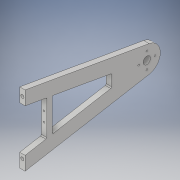
# Autodesk Inventor part: halter_seite
Saved by Autodesk Inventor 2017 (Build 210142000, 142)
## iProperties
Part Number: halter_seite
Material: Generisch
Document SubType Name: Modeling
Designer: Fabio
Density: 1 g/cm^3
Appearance: Vorgabe
Author: Fabio
Autodesk Inventor part; units mm, degrees
ref_plane "YZ Plane" through (0, 0, 0) normal (1, 0, 0) x (0, 1, 0)
ref_plane "XZ Plane" through (0, 0, 0) normal (0, 1, 0) x (-1, 0, 0)
ref_plane "XY Plane" through (0, 0, 0) normal (0, 0, 1) x (1, 0, 0)
sketch "Skizze1" plane through (0, 0, 0) normal (1, 0, 0) x (0, 1, 0)
  arc A0 (250, 65.0592) -> (229.3412, 89.6794) centre (225, 65.0592) ccw
  line L0 (225, 65.0592) -> (229.3412, 89.6794) construction
  line L1 (225, 65.0592) -> (250, 65.0592) construction
  line L2 (229.3412, 89.6794) -> (0, 130.1185)
  line L3 (0, 130.1185) -> (0, 104.7328)
  arc A1 (229.3412, 40.439) -> (250, 65.0592) centre (225, 65.0592) ccw
  line L4 (229.3412, 40.439) -> (0, 0)
  line L5 (0, 0) -> (92.864, 0) construction
  line L6 (0, 0) -> (0, 25.3857)
  line L7 (160, 76.5205) -> (160, 53.598)
  line L8 (40, 97.6797) -> (40, 32.4387)
  line L9 (50, 34.202) -> (50, 95.9165)
  line L10 (0, 104.7328) -> (40, 97.6797)
  line L11 (50, 95.9165) -> (160, 76.5205)
  line L12 (0, 25.3857) -> (40, 32.4387)
  line L13 (50, 34.202) -> (160, 53.598)
  dimension "d21" = 80
  dimension "d24" = 25
  dimension "d68" = 250
  dimension "d73" = 80
  dimension "d88" = 130.1185
  dimension "d89" = 79.3471
  dimension "d91" = 10
  dimension "d92" = 25
  dimension "d93" = 25
  dimension "d94" = 40
  dimension "d96" = 25
  dimension "d97" = 25
  dimension "d127" = 110
  constraints: 28 end point, 4 point on circle, 4 vertical, 2 centre point, 2 parallel, 2 symmetric about line, 1 coincident, 1 horizontal, 1 other
  measures "d21" angle of L1 L0
  measures "d24" radius of A0
  measures "d68" distance from line of L1.end L3
  measures "d73" angle of L3 L2
  measures "d88" distance of point (0, 0) L2.end
  measures "d89" distance of L6.end L3.end
  measures "d91" distance between parallel lines of L8 L9
  measures "d92" distance between parallel lines of L2 L11
  measures "d93" distance between parallel lines of L4 L13
  measures "d94" distance from line of L8 L3.end
  measures "d96" distance between parallel lines of L2 L10
  measures "d97" distance between parallel lines of L4 L12
  measures "d127" distance between parallel lines of L9 L7
extrude "Extrusion2" add sketch "Skizze1" along normal blind 10
sketch "Skizze7" plane through (10, 0, 0) normal (1, 0, 0) x (0, 0, -1)
  arc A0 (-40.439, 229.3412) -> (-89.6794, 229.3412) centre (-65.0592, 225) ccw projected
  point P0 (0, 0)
  constraints: 1 coincident
hole "Bohrung6" at (10, 225, 65.0592) direction (-1, 0, 0) diameter 13.6 end through all
sketch "Skizze8" plane through (10, 0, 0) normal (1, 0, 0) x (0, 0, -1)
  circle A0 centre (-65.0592, 225) radius 6.8 projected
  line L0 (-65.0592, 225) -> (-65.0592, 240) construction
  point P0 (0, 0)
  point P1 (-80.0592, 225)
  point P2 (-65.0592, 210)
  point P3 (-50.0592, 225)
  dimension "d107" = 15
  dimension "d110" = 360
  constraints: 2 end point, 1 coincident, 1 vertical, 5 other
  measures "d107" distance of L0.start L0.end
hole "Bohrung7" at (10, 240, 65.0592) at (10, 225, 80.0592) at (10, 210, 65.0592) at (10, 225, 50.0592) direction (-1, 0, 0) diameter 3 end through all
sketch "Skizze9" plane through (0, 0, 104.7328) normal (0, -1, 0) x (1, 0, 0)
  line L0 (0, 25.3857) -> (10, 25.3857) construction
  line L1 (5, 25.3857) -> (5, -104.7328) construction
  line L2 (0, -104.7328) -> (10, -104.7328) construction
  line L3 (0, 25.3857) -> (0, 0) construction
  line L4 (10, 25.3857) -> (10, 0) construction
  line L5 (0, 25.3857) -> (0, 0) construction
  line L6 (0, 0) -> (10, 0) construction
  line L7 (10, 25.3857) -> (10, 0) construction
  line L8 (0, 25.3857) -> (10, 25.3857) construction
  line L9 (0, 12.6928) -> (10, 12.6928) construction
  point P0 (5, 12.6928)
  point P1 (5, -87.3072)
  dimension "d119" = 100
  constraints: 5 midpoint, 4 end point, 1 point on line
  measures "d119" distance of point (5, 12.693) point (5, -87.307)
hole "Bohrung8" at (5, 0, 117.4256) at (5, 0, 17.4256) direction (0, 1, 0) diameter 6 depth 20 tip angle 118
sketch "Skizze10" plane through (0, 50, 95.9165) normal (0, 1, 0) x (1, 0, 0)
  line L0 (10, 61.7144) -> (10, 0) construction
  line L1 (10, 30.8572) -> (0, 30.8572) construction
  point P0 (0, 95.9165)
  point P1 (5, 21.8572)
  point P2 (5, 39.8572)
  dimension "d128" = 5
  dimension "d130" = 9
  dimension "d132" = 5
  dimension "d133" = 18
  constraints: 2 end point, 1 horizontal, 1 midpoint
  measures "d128" distance from line of point (5, 21.857) L0
  measures "d130" distance from line of L1 point (5, 21.857)
  measures "d132" distance from line of L0 point (5, 39.857)
  measures "d133" distance of point (5, 39.857) point (5, 21.857)
hole "Bohrung9" at (5, 50, 74.0592) at (5, 50, 56.0592) direction (0, -1, 0) diameter 3 end through all
fillet "Rundung1" radius 2 6 edges at (5, 160, 76.5205) (5, 40, 97.6797) (5, 50, 95.9165) (5, 50, 34.202) (5, 160, 53.598) (5, 40, 32.4387)
